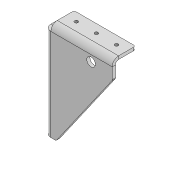
# Autodesk Inventor part: CCM_Mount_C
Saved by Autodesk Inventor 2020 (Build 240168000, 168)
## iProperties
Created: 2021-12-05
Part Number: CCM_Mount_C
Material: 一般
Document SubType Name: Sheet Metal
Designer: ken113
Density: 1 g/cm^3
Sheet Metal Rule: Default_mm
Appearance: 既定
Author: ken113
Autodesk Inventor part; units mm, degrees
ref_plane "YZ Plane" through (0, 0, 0) normal (1, 0, 0) x (0, 1, 0)
ref_plane "XZ Plane" through (0, 0, 0) normal (0, 1, 0) x (-1, 0, 0)
ref_plane "XY Plane" through (0, 0, 0) normal (0, 0, 1) x (1, 0, 0)
sketch "スケッチ1" plane through (0, 0, 0) normal (0, 0, 1) x (1, 0, 0)
  line L0 (29, -43.5) -> (-29, -43.5)
  line L1 (-29, -43.5) -> (-29, 43.5)
  line L2 (-29, 43.5) -> (29, 43.5)
  line L3 (29, 43.5) -> (29, -43.5)
  line L4 (29, -43.5) -> (-29, 43.5) construction
  line L5 (-29, -43.5) -> (29, 43.5) construction
  point P0 (0, 0)
  dimension "d0" = 87
  dimension "d1" = 58
  measures "d0" distance of L0.end L1.end
  measures "d1" distance of L1.end L2.end
extrude "プレート1" add sketch "スケッチ1" along normal blind 3
sketch "スケッチ2" plane through (-32, 43.5, -3) normal (-1, 0, 0) x (0, -1, 0)
  line L0 (87, 0) -> (0, 0)
  line L1 (0, 0) -> (0, -16)
  line L2 (0, -16) -> (87, -16)
  line L3 (87, -16) -> (87, 0)
  constraints: 6 end point, 1 horizontal, 1 perpendicular, 1 vertical
edge flange "フランジ1" height 22 angle 90 thickness 3 bend radius 3 thickness toward (-1, 0, 0) relief tear relief width 3 relief depth 1.5 edges at (-29, 0, 0) wall of the first edge with corners at (-32, -43.5, -3) (-32, 43.5, -3) (-32, 43.5, -19) (-32, -43.5, -19)
bend "曲げ1"
corner "コーナー1"
sketch "スケッチ3" plane through (29, 46.5, -3) normal (0, 1, 0) x (-1, 0, 0)
  line L0 (58, 0) -> (0, 0)
  line L1 (0, 0) -> (0, -16)
  line L2 (0, -16) -> (58, -16)
  line L3 (58, -16) -> (58, 0)
  constraints: 6 end point, 1 horizontal, 1 perpendicular, 1 vertical
edge flange "フランジ2" height 22 angle 90 thickness 3 bend radius 3 thickness toward (0, 1, 0) relief tear relief width 3 relief depth 1.5 edges at (0, 43.5, 0) wall of the first edge with corners at (-29, 46.5, -3) (29, 46.5, -3) (29, 46.5, -19) (-29, 46.5, -19)
bend "曲げ2"
corner "コーナー2"
sketch "スケッチ4" plane through (0, 0, 3) normal (0, 0, 1) x (1, 0, 0)
  line L0 (29, -43.5) -> (-29, -43.5) projected
  line L1 (-24, -43.5) -> (33.3099, 38.5)
  line L2 (-29, -43.5) -> (-29, 43.5) projected
  line L3 (-29, 43.5) -> (29, 43.5) projected
  line L4 (-29, -43.5) -> (-29, 43.5) projected
  line L5 (29, -43.5) -> (-29, -43.5) projected
  line L6 (29, 43.5) -> (29, -43.5) projected
  line L7 (-29, 43.5) -> (29, 43.5) projected
  point P0 (0, 0)
  point P1 (29, 32.3333)
  dimension "d23" = 5
  dimension "d24" = 5
  constraints: 2 end point, 1 point on line
  measures "d23" distance from line of L1.start L2
  measures "d24" distance from line of L3 L1.end
extrude "押し出し1" cut sketch "スケッチ4" against normal through all contours L0 L1 L6
fillet "フィレット1" radius 2 6 edges at (-24, -43.5, 1.5) (-33.5, -43.5, -19) (29, 32.3333, 1.5) (29, 48, -19) (-33.5, 43.5, -19) (-29, 48, -19)
sketch "スケッチ5" plane through (-32, -43.5, -3) normal (1, 0, 0) x (0, 0, -1)
  arc A0 (16, 85) -> (14, 87) centre (14, 85) ccw projected
  line L0 (14, 87) -> (0, 87) projected
  line L1 (0, 87) -> (0, 0) projected
  line L2 (14, 0) -> (0, 0) projected
  arc A1 (14, 0) -> (16, 2) centre (14, 2) ccw projected
  line L3 (16, 2) -> (16, 85) projected
  point P0 (-3, 43.5)
  point P1 (8, 77)
  point P2 (8, 10)
  point P3 (8, 43.5)
  dimension "d28" = 8
  dimension "d29" = 10
  dimension "d30" = 10
  dimension "d31" = 33.5
  constraints: 2 vertical alignment
  measures "d28" distance from line of L3 point (8, 77)
  measures "d29" distance from line of L0 point (8, 77)
  measures "d30" distance from line of point (8, 10) L2
  measures "d31" distance of point (8, 43.5) point (8, 10)
hole "穴1" at (-32, 33.5, -11) at (-32, -33.5, -11) at (-32, 0, -11) direction (-1, 0, 0) diameter 3.242 end through all thread size "M4x0.7" class "6H" standard "ISO Metric profile"
sketch "スケッチ6" plane through (-29, 49.5, -3) normal (0, 1, 0) x (1, 0, 0)
  line L0 (10, 8) -> (48, 8)
  line L1 (2, 16) -> (56, 16) projected
  line L2 (58, 14) -> (58, 0) projected
  line L3 (0, 0) -> (0, 14) projected
  point P0 (29, -3)
  point P1 (29, 8)
  dimension "d39" = 8
  dimension "d40" = 10
  dimension "d41" = 10
  constraints: 2 end point, 1 horizontal, 1 midpoint
  measures "d39" distance between parallel lines of L1 L0
  measures "d40" distance from line of L2 L0.end
  measures "d41" distance from line of L0.start L3
hole "穴2" at (0, 49.5, -11) at (19, 49.5, -11) at (-19, 49.5, -11) direction (0, -1, 0) diameter 3.242 end through all thread size "M4x0.7" class "6H" standard "ISO Metric profile"
sketch "スケッチ8" plane through (0, 0, 3) normal (0, 0, 1) x (1, 0, 0)
  line L0 (-29, 49.5) -> (29, 49.5) projected
  line L1 (29, 43.5) -> (29, 32.9629) projected
  point P0 (0, 0)
  point P1 (9, 37.5)
  dimension "d54" = 12
  dimension "d55" = 20
  measures "d54" distance from line of point (9, 37.5) L0
  measures "d55" distance from line of point (9, 37.5) L1
hole "穴3" at (9, 37.5, 3) direction (0, 0, -1) diameter 8.2 end through all
equation "\"d61\" = Thickness"
equation "\"d2\" = Thickness"
equation "\"d3\" = BendReliefWidth"
equation "\"d4\" = BendReliefDepth"
equation "\"d5\" = MinimumRemnant"
equation "\"d6\" = TransitionRadius"
equation "\"d9\" = BendRadius"
equation "\"d10\" = CornerReliefSize"
equation "\"d11\" = GapSize"
equation "\"d12\" = JacobiRadiusSize"
equation "\"d13\" = BendReliefWidth"
equation "\"d14\" = BendReliefDepth"
equation "\"d15\" = MinimumRemnant"
equation "\"d16\" = TransitionRadius"
equation "\"d19\" = BendRadius"
equation "\"d20\" = CornerReliefSize"
equation "\"d21\" = GapSize"
equation "\"d22\" = JacobiRadiusSize"
equation "\"BendRadius\" = Thickness"
equation "\"BendReliefWidth\" = Thickness"
equation "\"BendReliefDepth\" = 0.5 * Thickness"
equation "\"CornerReliefSize\" = 4 * Thickness"
equation "\"MinimumRemnant\" = 2 * Thickness"
equation "\"TransitionRadius\" = BendRadius"
equation "\"JacobiRadiusSize\" = BendRadius"
equation "\"GapSize\" = Thickness"
equation "\"Thickness\" = 3"
